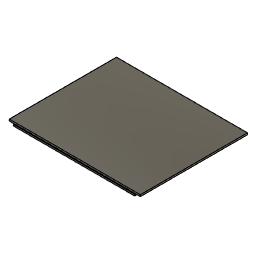
CoverPannel (Autodesk Fusion 360 design; units mm, degrees)
Autodesk Fusion 360 part; units mm, degrees
sketch "Sketch2" plane through (0, 0, 0) normal (0, 1, 0) x (1, 0, 0)
  line L0 (-71.8116, -9.5677) -> (91.1884, -9.5677)
  line L1 (91.1884, -9.5677) -> (91.1884, -7.5677)
  line L2 (91.1884, -7.5677) -> (-71.8116, -7.5677)
  line L3 (-71.8116, -7.5677) -> (-71.8116, -9.5677)
  line L4 (-78.3116, -11.7677) -> (97.6884, -11.7677)
  line L5 (97.6884, -11.7677) -> (97.6884, -9.5677)
  line L6 (97.6884, -9.5677) -> (-78.3116, -9.5677)
  line L7 (-78.3116, -9.5677) -> (-78.3116, -11.7677)
  dimension "d1" = 163
  dimension "d2" = 2
  dimension "d3" = 6.5
  dimension "d4" = 6.5
  dimension "d5" = 2.2
  constraint horizontal L0
  constraint vertical L1
  constraint horizontal L2
  constraint vertical L3
  constraint horizontal L4
  constraint vertical L5
  constraint horizontal L6
  constraint vertical L7
  constraint collinear L0 L6
  measures "d1" distance of L0.start L0.end
  measures "d2" distance of L0.start L2.end
  measures "d3" distance of L3 L7
  measures "d4" distance of L1 L5
  measures "d5" distance of L4.start L6.end
extrude "Extrude1" add sketch "Sketch2" along normal blind 145
extrude "Extrude2" cut sketch "Sketch2" along normal blind 1 contours L0 L4 L5 L6 L7
